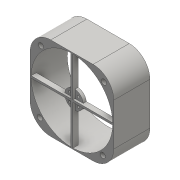
# Autodesk Inventor part: Motor mount (plain)
Saved by Autodesk Inventor 2016 (Build 200138000, 138)
## iProperties
Created: 2016-03-10
Part Number: Motor mount (plain)
Material: Generic
Document SubType Name: Modeling
Designer: s_sud
Density: 1 g/cm^3
Appearance: Default
Author: s_sud
Autodesk Inventor part; units mm, degrees
ref_plane "YZ Plane" through (0, 0, 0) normal (1, 0, 0) x (0, 1, 0)
ref_plane "XZ Plane" through (0, 0, 0) normal (0, 1, 0) x (-1, 0, 0)
ref_plane "XY Plane" through (0, 0, 0) normal (0, 0, 1) x (1, 0, 0)
sketch "Sketch1" plane through (0, 0, 0) normal (0, 1, 0) x (-1, 0, 0)
  circle A0 centre (0, 0) radius 39.5
  circle A1 centre (0, 0) radius 40.5
  dimension "d0" = 79
  dimension "d1" = 81
  constraints: 2 centre point, 2 coincident
  measures "d0" diameter of A0
  measures "d1" diameter of A1
extrude "Extrusion1" add sketch "Sketch1" along normal blind 35
sketch "Sketch12" plane through (0, 0, 0) normal (0, -1, 0) x (1, 0, 0)
  line L0 (-1, -40.5) -> (1, -40.5)
  line L1 (1, -40.5) -> (1, 40.5)
  line L2 (1, 40.5) -> (-1, 40.5)
  line L3 (-1, 40.5) -> (-1, -40.5)
  line L4 (-1, -40.5) -> (1, 40.5) construction
  line L5 (1, -40.5) -> (-1, 40.5) construction
  line L6 (-40.5, -1) -> (40.5, -1)
  line L7 (40.5, -1) -> (40.5, 1)
  line L8 (40.5, 1) -> (-40.5, 1)
  line L9 (-40.5, 1) -> (-40.5, -1)
  line L10 (-40.5, -1) -> (40.5, 1) construction
  line L11 (40.5, -1) -> (-40.5, 1) construction
  point P0 (0, 0)
  dimension "d64" = 81
  dimension "d65" = 2
  dimension "d66" = 81
  dimension "d67" = 2
  constraints: 24 end point, 4 midpoint, 4 parallel, 2 horizontal, 2 perpendicular
  measures "d64" distance of L0.end L1.end
  measures "d65" distance of L0.start L0.end
  measures "d66" distance of L7.end L8.end
  measures "d67" distance of L6.end L7.end
extrude "Extrusion12" add sketch "Sketch12" against normal blind 5
sketch "Sketch13" plane through (0, 5, 0) normal (0, 1, 0) x (1, 0, 0)
  circle A0 centre (0, 0) radius 9
  circle A1 centre (0, 6) radius 1
  circle A2 centre (-4.2426, 4.2426) radius 1
  circle A3 centre (-6, 0) radius 1
  circle A4 centre (-4.2426, -4.2426) radius 1
  circle A5 centre (0, -6) radius 1
  circle A6 centre (4.2426, -4.2426) radius 1
  circle A7 centre (6, 0) radius 1
  circle A8 centre (4.2426, 4.2426) radius 1
  dimension "d70" = 18
  dimension "d71" = 2
  dimension "d72" = 6
  dimension "d75" = 360
  constraints: 9 centre point, 1 coincident, 17 other
  measures "d70" diameter of A0
  measures "d71" diameter of A1
  measures "d72" distance of point (0, 0) A1.centre
extrude "Extrusion13" add sketch "Sketch13" against normal blind 3 contours A0 | A1 | A3 | A5 | A7
sketch "Sketch21" plane through (0, 35, 0) normal (0, 1, 0) x (1, 0, 0)
  line L0 (-40.5, -40.5) -> (40.5, -40.5)
  line L1 (40.5, -40.5) -> (40.5, 40.5)
  line L2 (40.5, 40.5) -> (-40.5, 40.5)
  line L3 (-40.5, 40.5) -> (-40.5, -40.5)
  line L4 (-40.5, -40.5) -> (40.5, 40.5) construction
  line L5 (40.5, -40.5) -> (-40.5, 40.5) construction
  circle A0 centre (0, 0) radius 40.5
  dimension "d111" = 81
  dimension "d112" = 81
  constraints: 12 end point, 2 midpoint, 2 parallel, 1 centre point, 1 coincident, 1 horizontal, 1 perpendicular, 1 tangent
  measures "d111" distance of L2.end L0.start
  measures "d112" distance of L0.start L0.end
extrude "Extrusion21" add sketch "Sketch21" against normal blind 35 contours L3 A0 L0 | A0 L1 L0 | L3 L2 A0 | A0 L2 L1
fillet "Fillet3" radius 20 4 edges at (-40.5, 17.5, -40.5) (40.5, 17.5, -40.5) (40.5, 17.5, 40.5) (-40.5, 17.5, 40.5)
sketch "Sketch23" plane through (0, 35, 0) normal (0, 1, 0) x (1, 0, 0)
  circle A0 centre (31, -31.0036) radius 2.5
  line L0 (0, 0) -> (0, -26.6326)
  line L1 (0, 0) -> (25.6096, -25.6096)
  circle A1 centre (29.9021, 31) radius 2.5
  circle A2 centre (-31, 29.9021) radius 2.5
  circle A3 centre (-29.9021, -31) radius 2.5
  line L2 (25.6096, -25.6096) -> (31.7098, -31.7098)
  dimension "d123" = 5
  dimension "d124" = 45
  dimension "d125" = 31
  dimension "d128" = 360
  constraints: 6 end point, 4 centre point, 2 coincident, 1 vertical, 7 other
  measures "d123" diameter of A0
  measures "d124" angle of L0 L1
  measures "d125" horizontal distance of L0.start A0.centre
extrude "Extrusion23" cut sketch "Sketch23" against normal blind 100
body "Solid1"
